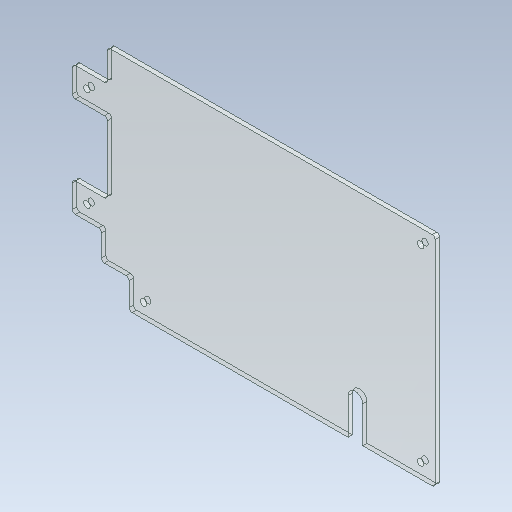
# Autodesk Inventor part: SideAcrylicSheet
Saved by Autodesk Inventor 2021 (Build 250183000, 183)
## iProperties
Created: 2020-07-16
Part Number: SideAcrylicSheet
Material: Generic
Document SubType Name: Modeling
Designer: CASE-SMALL2
Density: 1 g/cm^3
Appearance: Default
Author: CASE-SMALL2
Autodesk Inventor part; units mm, degrees
ref_plane "YZ Plane" through (0, 0, 0) normal (1, 0, 0) x (0, 1, 0)
ref_plane "XZ Plane" through (0, 0, 0) normal (0, 1, 0) x (-1, 0, 0)
ref_plane "XY Plane" through (0, 0, 0) normal (0, 0, 1) x (1, 0, 0)
sketch "Sketch1" plane through (0, 0, 0) normal (0, 0, 1) x (1, 0, 0)
  line L0 (-125, -75) -> (125, -75)
  line L1 (125, -75) -> (125, 75)
  line L2 (125, 75) -> (-125, 75)
  line L3 (-125, 75) -> (-125, -75)
  line L4 (-125, -75) -> (125, 75) construction
  line L5 (125, -75) -> (-125, 75) construction
  point P0 (0, 0)
  dimension "d0" = 150
  dimension "d1" = 250
  constraints: 12 end point, 2 midpoint, 2 parallel, 1 horizontal, 1 perpendicular
  measures "d0" distance of L2.end L0.start
  measures "d1" distance of L1.end L2.end
extrude "Extrusion1" add sketch "Sketch1" along normal blind 3
sketch "Sketch2" plane through (0, 0, 3) normal (0, 0, 1) x (1, 0, 0)
  line L0 (125, -75) -> (125, 75) construction
  line L1 (125, 75) -> (-125, 75) construction
  line L2 (-125, 75) -> (-125, -75) construction
  line L3 (-125, -75) -> (125, -75) construction
  line L4 (-125, -36) -> (-105, -36)
  line L5 (-105, -36) -> (-105, -55)
  line L6 (-105, -55) -> (-86, -55)
  line L7 (-86, -55) -> (-86, -75)
  line L8 (-125, -75) -> (125, -75) construction
  line L9 (-125, 75) -> (-125, -75) construction
  line L10 (-125, -36) -> (-125, -75)
  line L11 (-86, -75) -> (-125, -75)
  line L12 (-125, 33) -> (-101, 33)
  line L13 (-101, 33) -> (-101, -16)
  line L14 (-101, -16) -> (-125, -16)
  line L15 (-125, -16) -> (-125, 33)
  line L16 (65, -75) -> (75, -75)
  line L17 (75, -75) -> (75, -45)
  line L18 (75, -45) -> (65, -45)
  line L19 (65, -45) -> (65, -75)
  line L20 (125, 75) -> (-125, 75) projected
  line L21 (-125, 75) -> (-101, 75)
  line L22 (-101, 75) -> (-101, 53)
  line L23 (-101, 53) -> (-125, 53)
  line L24 (-125, 53) -> (-125, 75)
  point P0 (0, 0)
  dimension "d4" = 39
  dimension "d5" = 39
  dimension "d6" = 20
  dimension "d7" = 20
  dimension "d9" = 24
  dimension "d11" = 20
  dimension "d13" = 10
  dimension "d14" = 30
  dimension "d36" = 50
  dimension "d37" = 22
  dimension "d39" = 42
  constraints: 36 end point, 7 perpendicular, 6 parallel, 4 point on line, 3 horizontal, 2 collinear
  measures "d4" distance between parallel lines of L7 L2
  measures "d5" distance between parallel lines of L3 L4
  measures "d6" distance between parallel lines of L5 L2
  measures "d7" distance between parallel lines of L3 L6
  measures "d9" distance between parallel lines of L15 L13
  measures "d11" distance between parallel lines of L4 L14
  measures "d13" distance between parallel lines of L17 L19
  measures "d14" distance between parallel lines of L3 L18
  measures "d36" distance between parallel lines of L0 L17
  measures "d37" distance between parallel lines of L21 L23
  measures "d39" distance between parallel lines of L1 L12
extrude "Extrusion2" cut sketch "Sketch2" against normal blind 3
sketch "Sketch3" plane through (0, 0, 3) normal (0, 0, 1) x (1, 0, 0)
  circle A0 centre (-115, 43) radius 2.25
  circle A1 centre (-115, -26) radius 2.25
  circle A2 centre (115, 65) radius 2.25
  circle A3 centre (115, -65) radius 2.25
  circle A4 centre (-76, -65) radius 2.25
  line L0 (125, 75) -> (-125, 75) projected
  line L1 (-125, 75) -> (-125, 33) projected
  line L2 (-125, -16) -> (-125, -36) projected
  line L3 (-125, -36) -> (-105, -36) projected
  line L4 (-86, -75) -> (65, -75) projected
  line L5 (-86, -55) -> (-86, -75) projected
  line L6 (75, -75) -> (125, -75) projected
  line L7 (125, -75) -> (125, 75) projected
  line L8 (-125, 53) -> (-101, 53) projected
  point P0 (0, 0)
  dimension "d17" = 4.5
  dimension "d18" = 4.5
  dimension "d19" = 4.5
  dimension "d20" = 4.5
  dimension "d21" = 4.5
  dimension "d23" = 10
  dimension "d24" = 10
  dimension "d25" = 10
  dimension "d26" = 10
  dimension "d27" = 10
  dimension "d28" = 10
  dimension "d29" = 10
  dimension "d30" = 10
  dimension "d31" = 10
  dimension "d38" = 10
  constraints: 5 centre point
  measures "d17" diameter of A0
  measures "d18" diameter of A1
  measures "d19" diameter of A4
  measures "d20" diameter of A3
  measures "d21" diameter of A2
  measures "d23" distance from line of L1 A0.centre
  measures "d24" distance from line of L2 A1.centre
  measures "d25" distance from line of L3 A1.centre
  measures "d26" distance from line of L4 A4.centre
  measures "d27" distance from line of L5 A4.centre
  measures "d28" distance from line of L6 A3.centre
  measures "d29" distance from line of L7 A3.centre
  measures "d30" distance from line of L7 A2.centre
  measures "d31" distance from line of L0 A2.centre
  measures "d38" distance from line of L8 A0.centre
extrude "Extrusion3" cut sketch "Sketch3" against normal through all
fillet "Fillet1" radius 2 14 edges at (125, 75, 1.5) (125, -75, 1.5) (-86, -75, 1.5) (-86, -55, 1.5) (-105, -55, 1.5) (-105, -36, 1.5) (-125, -36, 1.5) (-125, -16, 1.5) (-101, -16, 1.5) (-101, 33, 1.5) (-125, 33, 1.5) (-125, 53, 1.5) (-101, 53, 1.5) (-101, 75, 1.5)
fillet "Fillet1" radius 5 2 edges at (65, -45, 1.5) (75, -45, 1.5)
sketch "Sketch4" plane through (0, 0, 3) normal (0, 0, 1) x (1, 0, 0)
  arc A0 (-99, 75) -> (-101, 73) centre (-99, 73) ccw projected
  line L0 (-101, 73) -> (-101, 55) projected
  arc A1 (-103, 53) -> (-101, 55) centre (-103, 55) ccw projected
  line L1 (-103, 53) -> (-123, 53) projected
  arc A2 (-123, 53) -> (-125, 51) centre (-123, 51) ccw projected
  line L2 (-125, 51) -> (-125, 35) projected
  arc A3 (-125, 35) -> (-123, 33) centre (-123, 35) ccw projected
  line L3 (-123, 33) -> (-103, 33) projected
  arc A4 (-101, 31) -> (-103, 33) centre (-103, 31) ccw projected
  line L4 (-101, 31) -> (-101, -14) projected
  arc A5 (-103, -16) -> (-101, -14) centre (-103, -14) ccw projected
  line L5 (-103, -16) -> (-123, -16) projected
  arc A6 (-123, -16) -> (-125, -18) centre (-123, -18) ccw projected
  line L6 (-125, -18) -> (-125, -34) projected
  arc A7 (-125, -34) -> (-123, -36) centre (-123, -34) ccw projected
  line L7 (-123, -36) -> (-107, -36) projected
  arc A8 (-105, -38) -> (-107, -36) centre (-107, -38) ccw projected
  line L8 (-105, -38) -> (-105, -53) projected
  arc A9 (-105, -53) -> (-103, -55) centre (-103, -53) ccw projected
  line L9 (-103, -55) -> (-88, -55) projected
  arc A10 (-86, -57) -> (-88, -55) centre (-88, -57) ccw projected
  line L10 (-86, -57) -> (-86, -73) projected
  arc A11 (-86, -73) -> (-84, -75) centre (-84, -73) ccw projected
  line L11 (-84, -75) -> (65, -75) projected
  line L12 (65, -75) -> (65, -50) projected
  arc A12 (75, -50) -> (65, -50) centre (70, -50) ccw projected
  line L13 (75, -50) -> (75, -75) projected
  line L14 (75, -75) -> (123, -75) projected
  arc A13 (123, -75) -> (125, -73) centre (123, -73) ccw projected
  line L15 (125, -73) -> (125, 73) projected
  arc A14 (125, 73) -> (123, 75) centre (123, 73) ccw projected
  line L16 (123, 75) -> (-99, 75) projected
  circle A15 centre (-115, 43) radius 2.25 projected
  circle A16 centre (115, 65) radius 2.25 projected
  circle A17 centre (-115, -26) radius 2.25 projected
  circle A18 centre (115, -65) radius 2.25 projected
  circle A19 centre (-76, -65) radius 2.25 projected
  point P0 (0, 0)
equation "\"d5\" = d4"
equation "\"d18\" = d17"
equation "\"d19\" = d17"
equation "\"d20\" = d17"
equation "\"d21\" = d17"
equation "\"d24\" = d23"
equation "\"d25\" = d23"
equation "\"d26\" = d25"
equation "\"d27\" = d25"
equation "\"d28\" = d26"
equation "\"d29\" = d26"
equation "\"d30\" = d23"
equation "\"d31\" = d23"
equation "\"d38\" = d23"
body "Solid1"
